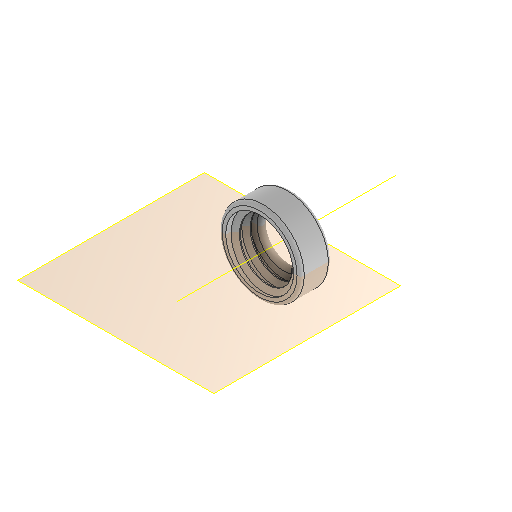
# Autodesk Inventor part: 20_Cube_4_insert_Photosensor_lenscap
Saved by Autodesk Inventor 2025.1 (Build 291241020, 241B)
## iProperties
Created: 2024-10-04
Part Number: 20_Cube_4_insert_Photosensor_lenscap
Material: Generic
Document SubType Name: Modeling
Designer: diederichbenedict
Density: 1 g/cm^3
Appearance: Default
Author: diederichbenedict
Autodesk Inventor part; units mm, degrees
ref_plane "YZ Plane" through (0, 0, 0) normal (1, 0, 0) x (0, 1, 0)
ref_plane "XZ Plane" through (0, 0, 0) normal (0, 1, 0) x (-1, 0, 0)
ref_plane "XY Plane" through (0, 0, 0) normal (0, 0, 1) x (1, 0, 0)
ref_plane "Work Plane1" through (0, 46.8, 0) normal (0, 0, 1) x (-1, 0, 0)
sketch "Sketch2" plane through (0, 46.8, 0) normal (0, 0, 1) x (-1, 0, 0)
  spline S0 degree 3 number of poles 148
  spline S1 degree 3 number of poles 148
  line L0 (31.3425, -5.6798) -> (32.5946, -4.8031)
  line L1 (32.5946, -4.1553) -> (31.3425, -3.2786)
  line L2 (31.3425, -3.2786) -> (31.3425, -5.6037)
  line L3 (32.5946, -4.8031) -> (32.5946, -4.1553)
  line L4 (31.3425, 13.5614) -> (31.3425, -5.6037)
  line L5 (32.8425, -4.1071) -> (31.4425, -3.1268)
  line L6 (31.4425, -3.1268) -> (31.4425, -2.831)
  line L7 (31.4425, -2.831) -> (32.8425, -1.8994)
  line L8 (32.8425, -1.8994) -> (32.8425, -4.1071)
  point P0 (0, 46.8)
  point P1 (31.9686, -3.7169)
  point P2 (32.1425, -3.6169)
  point P3 (31.4425, -2.9789)
  dimension "d4" = 0
  dimension "d5" = 0.1
  dimension "d6" = 0.1
  dimension "d7" = 1.4
  constraints: 10 end point, 3 midpoint, 2 vertical, 1 parallel, 1 other
  measures "d4" angle of L1 L5
  measures "d5" vertical distance of point (31.969, -3.717) point (32.143, -3.617)
  measures "d6" distance from line of L4 point (31.443, -2.979)
  measures "d7" distance from line of point (31.443, -2.979) L8
coil "Coil1" sketch "Sketch2" operation add axis through (-23.4, 35.1998, 0) along (0, -1, 0) pitch 3 turns 2.5 hand right contours L5 L6 L7 L8
sketch "Sketch3" plane through (0, 46.8, 0) normal (0, 0, 1) x (-1, 0, 0)
  line L0 (13.9575, 5.6006) -> (13.9575, 3.3929) projected
  line L1 (32.8425, -1.8994) -> (32.8425, -4.1071) projected
  line L2 (15.3575, 4.669) -> (13.9575, 5.6006) projected
  line L3 (13.9575, 5.6006) -> (11.9575, 5.6006)
  line L4 (11.9575, 5.6006) -> (11.9575, -1.1071)
  line L5 (11.9575, -1.1071) -> (13.9575, -1.1071)
  line L6 (13.9575, -1.1071) -> (13.9575, 5.6006)
  line L7 (11.9575, -1.1071) -> (16.9575, -1.1071)
  line L8 (16.9575, -1.1071) -> (16.9575, -3.1071)
  line L9 (16.9575, -3.1071) -> (11.9575, -3.1071)
  line L10 (11.9575, -3.1071) -> (11.9575, -1.1071)
  line L11 (23.4, 56.7814) -> (23.4, -13.0885) projected
  point P0 (0, 46.8)
  dimension "d16" = 2
  dimension "d17" = 5
  dimension "d18" = 2
  constraints: 16 end point, 4 parallel, 2 horizontal, 2 perpendicular
  measures "d16" distance of L5.end L4.end
  measures "d17" distance of L8.end L9.end
  measures "d18" distance of L7.end L8.end
revolve "Revolution2" add sketch "Sketch3" angle 360 about axis through (-23.4, 35.1998, 0) along (0, 1, 0)
fillet "Fillet1" radius 1 4 edges at (-34.8425, 49.9071, 0) (-29.8425, 49.9071, 0) (-29.8425, 47.9071, 0) (-34.8425, 41.1994, 0)
body "Solid2"
